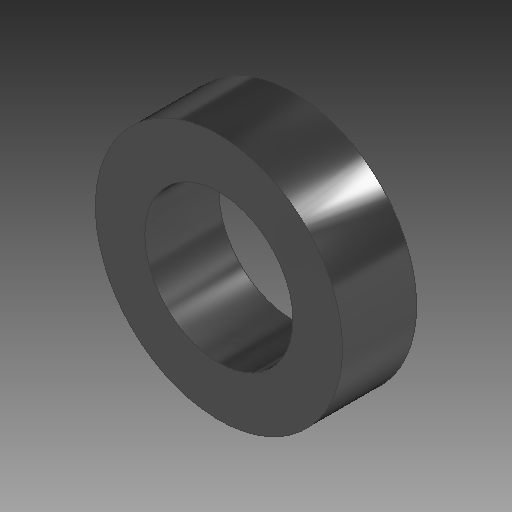
# Autodesk Inventor part: オイレス グライトロン0610,3t
Saved by Autodesk Inventor 2020 (Build 240168000, 168)
## iProperties
Created: 2019-07-24
Part Number: オイレス グライトロン0610,3t
Material: ポリテトラフルオロエチレン
Document SubType Name: Modeling
Designer: 雪村
Mass: 0.304609 g
Surface Area: 2.51327 cm^2
Volume: 0.150796 cm^3
Density: 2.02 g/cm^3
Appearance: ラッカー - 黒
Author: 雪村
Autodesk Inventor part; units mm, degrees
ref_plane "YZ Plane" through (0, 0, 0) normal (1, 0, 0) x (0, 1, 0)
ref_plane "XZ Plane" through (0, 0, 0) normal (0, 1, 0) x (-1, 0, 0)
ref_plane "XY Plane" through (0, 0, 0) normal (0, 0, 1) x (1, 0, 0)
sketch "スケッチ1" plane through (0, 0, 0) normal (0, 0, 1) x (1, 0, 0)
  circle A0 centre (0, 0) radius 3
  circle A1 centre (0, 0) radius 5
  dimension "d0" = 6
  dimension "d1" = 10
  constraints: 2 centre point, 2 coincident
  measures "d0" diameter of A0
  measures "d1" diameter of A1
extrude "押し出し1" add sketch "スケッチ1" along normal blind 3
